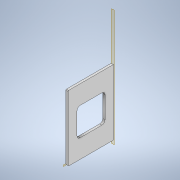
# Autodesk Inventor part: cover_components
Saved by Autodesk Inventor 2020 (Build 240168000, 168)
## iProperties
Created: 2020-01-09
Part Number: cover_components
Material: Generic
Document SubType Name: Modeling
Designer: erwin
Density: 1 g/cm^3
Appearance: Default
Author: erwin
Autodesk Inventor part; units mm, degrees
ref_plane "YZ Plane" through (0, 0, 0) normal (1, 0, 0) x (0, 1, 0)
ref_plane "XZ Plane" through (0, 0, 0) normal (0, 1, 0) x (-1, 0, 0)
ref_plane "XY Plane" through (0, 0, 0) normal (0, 0, 1) x (1, 0, 0)
ref_plane "Work Plane1" through (0, 0, 0) normal (0, 0, 1) x (1, 0, 0)
ref_plane "Work Plane2" through (0, -170, 73.6) normal (1, 0, 0) x (0, 0, 1)
sketch "Sketch2" plane through (0, -170, 73.6) normal (1, 0, 0) x (0, 0, 1)
  line L0 (-73.6, -170) -> (-73.6, 0) projected
  line L1 (0, 1.8) -> (-73.6, 1.8)
  line L2 (-73.6, 1.8) -> (-73.6, -103.2)
  line L3 (-73.6, -103.2) -> (0, -103.2)
  line L4 (0, -103.2) -> (0, 1.8)
  dimension "d0" = 105
  constraints: 8 end point, 2 parallel, 1 horizontal, 1 perpendicular, 1 point on line, 1 other
  measures "d0" distance of L2.end L1.end
extrude "Extrusion1" add sketch "Sketch2" along normal blind 3.6
sketch "Sketch3" plane through (3.6, -170, 73.6) normal (1, 0, 0) x (0, 0, -1)
  line L0 (73.6, -1.8) -> (73.6, 103.2) projected
  line L1 (73.6, 103.2) -> (0, 103.2) projected
  line L2 (0, 103.2) -> (0, -1.8) projected
  line L3 (0, -1.8) -> (73.6, -1.8) projected
  line L4 (73.6, 103.2) -> (0, 103.2) construction
  line L5 (73.6, -1.8) -> (73.6, 103.2) construction
  line L6 (36.8, 103.2) -> (73.6, 103.2) construction
  line L7 (73.6, 103.2) -> (73.6, 50.7) construction
  line L8 (73.6, 50.7) -> (36.8, 50.7) construction
  line L9 (36.8, 50.7) -> (36.8, 103.2) construction
  line L10 (19.3, 28.2) -> (54.3, 28.2)
  line L11 (59.3, 33.2) -> (59.3, 68.2)
  line L12 (54.3, 73.2) -> (19.3, 73.2)
  line L13 (14.3, 68.2) -> (14.3, 33.2)
  line L14 (14.3, 28.2) -> (59.3, 73.2) construction
  line L15 (59.3, 28.2) -> (14.3, 73.2) construction
  arc A0 (19.3, 73.2) -> (14.3, 68.2) centre (19.3, 68.2) ccw
  arc A1 (59.3, 68.2) -> (54.3, 73.2) centre (54.3, 68.2) ccw
  arc A2 (54.3, 28.2) -> (59.3, 33.2) centre (54.3, 33.2) ccw
  arc A3 (14.3, 33.2) -> (19.3, 28.2) centre (19.3, 33.2) ccw
  point P0 (73.6, 170)
  dimension "d3" = 45
  dimension "d4" = 45
  dimension "d5" = 5
  constraints: 20 end point, 8 point on circle, 8 point on line, 8 tangent, 4 centre point, 4 midpoint, 4 parallel, 3 equal radius, 2 horizontal, 2 perpendicular
  measures "d3" distance of L15.end L14.end
  measures "d4" distance of L14.end L15.start
  measures "d5" radius of A0
extrude "Extrusion2" cut sketch "Sketch3" against normal through all contours A3 L13 A0 L12 A1 L11 A2 L10
chamfer "Chamfer1" distance 1 angle 45 4 edges at (1.8, -66.8, 73.6) (1.8, -171.8, 73.6) (1.8, -66.8, 0) (1.8, -171.8, 0)
equation "\"d1\" = wood_thickness"
equation "\"wood_thickness\" = 3.6"
body "Solid1"
